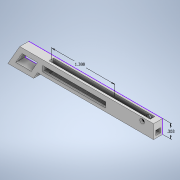
# Autodesk Inventor part: Crossbow holder
Saved by Autodesk Inventor 2021 (Build 250183000, 183)
## iProperties
Created: 2020-07-07
Part Number: Crossbow holder
Material: Generic
Document SubType Name: Modeling
Designer: saipr
Density: 1 g/cm^3
Appearance: Default
Author: saipr
Autodesk Inventor part; units mm, degrees
ref_plane "YZ Plane" through (0, 0, 0) normal (1, 0, 0) x (0, 1, 0)
ref_plane "XZ Plane" through (0, 0, 0) normal (0, 1, 0) x (-1, 0, 0)
ref_plane "XY Plane" through (0, 0, 0) normal (0, 0, 1) x (1, 0, 0)
sketch "Sketch1" plane through (0, 0, 0) normal (0, 0, 1) x (1, 0, 0)
  line L0 (0, 0) -> (3.4799, 6.0274)
  line L1 (3.4799, 6.0274) -> (12.1665, 6.0274)
  line L2 (0, 0) -> (8.6866, 0)
  line L3 (8.6866, 0) -> (12.1665, 6.0274)
  line L4 (-4.4376, -2.7527) -> (2.2208, 8.7801)
  line L5 (2.2208, 8.7801) -> (16.6041, 8.7801)
  line L6 (-4.4376, -2.7527) -> (9.9456, -2.7527)
  line L7 (9.9456, -2.7527) -> (12.1665, 1.0938)
  line L8 (12.1665, 1.0938) -> (77.0093, 1.0938)
  line L9 (77.0093, 1.0938) -> (77.0093, 8.7801)
  line L10 (77.0093, 8.7801) -> (12.1665, 8.7801)
  line L11 (15.0148, 6.0274) -> (50.27, 6.0274)
  line L12 (50.27, 6.0274) -> (50.27, 3.0137)
  line L13 (50.27, 3.0137) -> (15.0148, 3.0137)
  line L14 (15.0148, 3.0137) -> (15.0148, 6.0274)
  dimension "d29" = 7.6862
  dimension "d48" = 35.2552
  constraints: 30 end point, 9 parallel, 2 point on line, 1 horizontal, 1 perpendicular
  measures "d29" distance of L8.end L9.end
  measures "d48" distance of L11.start L11.end
extrude "Extrusion1" add sketch "Sketch1" along normal blind 5.08 contours L4 L5 L10 L9 L8 L7 L6 | L11 L12 L13 L14
sketch "Sketch2" plane through (0, 0, 5.08) normal (0, 0, 1) x (1, 0, 0)
  line L0 (77.0093, 8.7801) -> (2.2208, 8.7801) projected
  line L1 (77.0093, 8.7801) -> (70.6593, 8.7801)
  line L2 (70.6593, 8.7801) -> (70.6593, 4.9701)
  circle A0 centre (70.6593, 6.8751) radius 1.27
  point P0 (0, 0)
  dimension "d30" = 6.35
  dimension "d31" = 3.81
  dimension "d32" = 2.54
  constraints: 4 end point, 1 centre point, 1 midpoint, 1 perpendicular, 1 point on line
  measures "d30" distance of L0.start L1.end
  measures "d31" distance of L1.end L2.end
  measures "d32" diameter of A0
hole "Hole1" at (70.6593, 6.8751, 5.08) direction (0, 0, -1) diameter 2.54 end through all
sketch "Sketch3" plane through (2.2208, 8.7801, 0) normal (0, 1, 0) x (1, 0, 0)
  line L0 (71.6928, -2.54) -> (71.6928, -1.27)
  line L1 (71.6928, -1.27) -> (71.6928, -3.81)
  line L2 (71.6928, -3.81) -> (15.0985, -3.81)
  line L3 (15.0985, -3.81) -> (15.0985, -1.27)
  line L4 (15.0985, -1.27) -> (71.6928, -1.27)
  point P0 (-2.2208, 0)
  dimension "d40" = 1.27
  dimension "d41" = 2.54
  constraints: 10 end point, 2 parallel, 1 perpendicular
  measures "d40" distance of L0.start L0.end
  measures "d41" distance of L0.end L1.end
extrude "Extrusion2" cut sketch "Sketch3" against normal blind 6.35
sketch "Sketch4" plane through (77.0093, 1.0938, 0) normal (1, 0, 0) x (0, 0, -1)
  line L0 (-1.27, 7.6862) -> (-1.27, 1.3362) projected
  line L1 (-3.81, 7.6862) -> (-3.81, 1.3362) projected
  line L2 (-1.27, 1.3362) -> (-3.81, 1.3362)
  line L3 (-3.81, 1.3362) -> (-3.81, 3.8762)
  line L4 (-3.81, 3.8762) -> (-1.27, 3.8762)
  line L5 (-1.27, 3.8762) -> (-1.27, 1.3362)
  point P0 (0, -1.0938)
  dimension "d45" = 2.54
  constraints: 8 end point, 2 parallel, 2 perpendicular
  measures "d45" distance of L1.end L3.end
extrude "Extrusion3" cut sketch "Sketch4" against normal blind 8.89
extrude "Extrusion4" cut sketch "Sketch1" along normal blind 5.08 contours L11 L12 L13 L14
body "Solid1"
